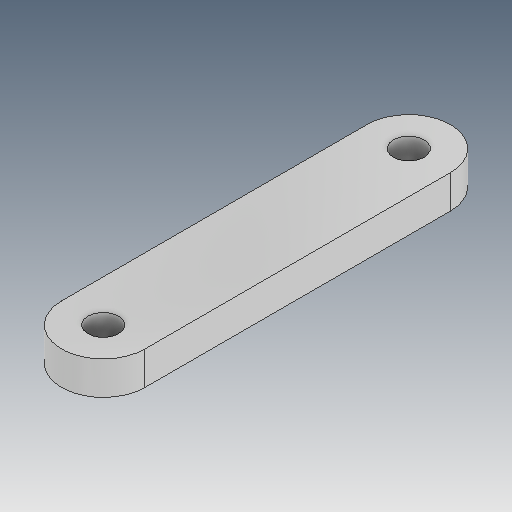
# Autodesk Inventor part: BaseTensionBracket
Saved by Autodesk Inventor 2020.3 (Build 243373000, 373)
## iProperties
Created: 2021-10-18
Part Number: BaseTensionBracket
Material: Aluminum 6061
Document SubType Name: Modeling
Designer: justi
Density: 2.7 g/cm^3
Appearance: Aluminum - Polished
Mass: 15.458 g
Surface Area: 30.5848 cm^2
Volume: 5.72519 cm^3
Author: justi
Autodesk Inventor part; units mm, degrees
ref_plane "YZ Plane" through (0, 0, 0) normal (1, 0, 0) x (0, 1, 0)
ref_plane "XZ Plane" through (0, 0, 0) normal (0, 1, 0) x (-1, 0, 0)
sketch "Sketch1" plane through (0, 0, 0) normal (0, 1, 0) x (-1, 0, 0)
  circle A0 centre (0, 0) radius 2.75
  line L0 (0, 0) -> (0, -55) construction
  circle A1 centre (0, -55) radius 2.75
  line L1 (0, 0) -> (0, -55) construction
  line L2 (-7.5, 0) -> (-7.5, -55)
  line L3 (7.5, -55) -> (7.5, 0)
  arc A2 (7.5, 0) -> (-7.5, 0) centre (0, 0) ccw
  arc A3 (-7.5, -55) -> (7.5, -55) centre (0, -55) ccw
  point P0 (0, -27.5)
  dimension "d0" = 5.5
  dimension "d1" = 55
  dimension "d2" = 5.5
  dimension "d3" = 15
  constraints: 10 end point, 4 centre point, 4 point on circle, 4 tangent, 2 coincident, 2 equal length, 2 midpoint, 1 vertical
  measures "d0" diameter of A0
  measures "d1" distance of L0.start L0.end
  measures "d2" diameter of A1
  measures "d3" diameter of A3
extrude "Extrusion1" add sketch "Sketch1" along normal blind 6
ref_plane "Work Plane1" through (0, 0, -27.5) normal (0, 0, 1) x (1, 0, 0)
body "Solid1"
